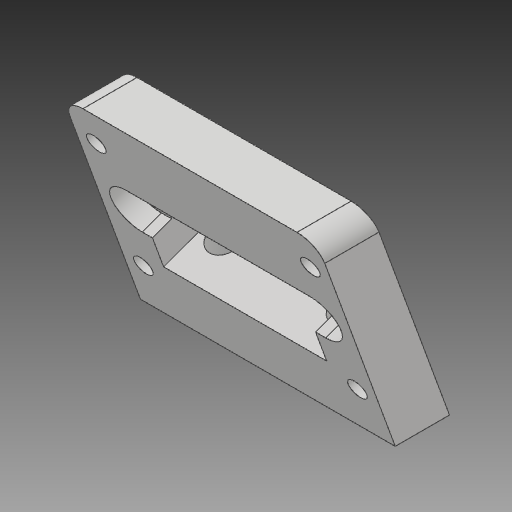
# Autodesk Inventor part: Kamerahalter Vorne geneigt
Saved by Autodesk Inventor 2019.4 (Build 234330000, 330)
## iProperties
Part Number: Kamerahalter Vorne geneigt
Material: Generisch
Document SubType Name: Modeling
Designer: rYan
Density: 1 g/cm^3
Appearance: Vorgabe
Mass: 1.96506 g
Surface Area: 17.9006 cm^2
Volume: 1.96506 cm^3
Author: rYan
Autodesk Inventor part; units mm, degrees
ref_plane "YZ Plane" through (0, 0, 0) normal (1, 0, 0) x (0, 1, 0)
ref_plane "XZ Plane" through (0, 0, 0) normal (0, 1, 0) x (-1, 0, 0)
ref_plane "XY Plane" through (0, 0, 0) normal (0, 0, 1) x (1, 0, 0)
sketch "Skizze1" plane through (0, 0, 0) normal (1, 0, 0) x (0, 1, 0)
  line L0 (2.6604, 0) -> (-2.6604, 0)
  line L1 (-2.6604, 0) -> (-10.3038, 21)
  line L2 (-10.3038, 21) -> (-4.9829, 21)
  line L3 (-4.9829, 21) -> (2.6604, 0)
  point P0 (0, 0)
  point P1 (0, 0)
  dimension "d1" = 21
  dimension "d2" = 70
  dimension "d33" = 5
  constraints: 8 end point, 2 parallel, 1 coincident, 1 horizontal, 1 midpoint
  measures "d1" distance between parallel lines of L0 L2
  measures "d2" angle of L0 L1
  measures "d33" distance between parallel lines of L3 L1
extrude "Extrusion1" add sketch "Skizze1" along normal mid plane 25
sketch "Skizze3" plane through (-12.5, -2.6604, 0) normal (0, -0.9396926, -0.3420201) x (1, 0, 0)
  line L0 (25, 0) -> (0, 0) projected
  line L1 (25, 22.3477) -> (25, 0) projected
  line L2 (25, 22.3477) -> (0, 22.3477) projected
  line L3 (0, 0) -> (0, 22.3477) projected
  line L4 (3.5, 12) -> (21.5, 12) construction
  line L5 (3.5, 9.7) -> (21.5, 9.7)
  line L6 (21.5, 14.3) -> (3.5, 14.3)
  arc A0 (3.5, 14.3) -> (3.5, 9.7) centre (3.5, 12) ccw
  arc A1 (21.5, 9.7) -> (21.5, 14.3) centre (21.5, 12) ccw
  line L7 (12.5, 22.3477) -> (12.5, 0) construction
  point P0 (12.5, -0.9099)
  point P1 (12.5, 12)
  dimension "d10" = 4.6
  dimension "d11" = 18
  dimension "d12" = 12
  constraints: 10 end point, 4 point on circle, 4 tangent, 3 midpoint, 2 centre point, 1 horizontal, 1 parallel, 1 point on line
  measures "d10" diameter of A1
  measures "d11" distance of L4.start L4.end
  measures "d12" distance between parallel lines of L0 L4
extrude "Extrusion3" cut sketch "Skizze3" against normal blind 2 contours A0 L6 A1 L5
sketch "Skizze4" plane through (-12.5, -2.6604, 0) normal (0, -0.9396926, -0.3420201) x (1, 0, 0)
  line L0 (2, 18.5) -> (23, 18.5) construction
  line L1 (23, 18.5) -> (23, 5) construction
  line L2 (23, 5) -> (2, 5) construction
  line L3 (2, 5) -> (2, 18.5) construction
  line L4 (3.5, 14.3) -> (21.5, 14.3) projected
  arc A0 (21.5, 9.7) -> (21.5, 14.3) centre (21.5, 12) ccw projected
  line L5 (21.5, 9.7) -> (3.5, 9.7) projected
  arc A1 (3.5, 14.3) -> (3.5, 9.7) centre (3.5, 12) ccw projected
  line L6 (25, 0) -> (0, 0) projected
  line L7 (25, 22.3477) -> (25, 0) projected
  line L8 (25, 22.3477) -> (0, 22.3477) projected
  line L9 (0, 0) -> (0, 22.3477) projected
  line L10 (25, 22.3477) -> (0, 22.3477) construction
  line L11 (12.5, 22.3477) -> (12.5, 0) construction
  line L12 (25, 0) -> (0, 0) construction
  point P0 (12.5, -0.9099)
  dimension "d15" = 21
  dimension "d16" = 13.5
  dimension "d34" = 7
  constraints: 10 end point, 4 coincident, 2 midpoint, 2 parallel, 1 horizontal, 1 perpendicular, 1 other
  measures "d15" distance of L0.start L0.end
  measures "d16" distance of L2.end L0.start
  measures "d34" distance from line of L2 A1.centre
hole "Bohrung1" at (-10.5, -8.9878, 17.3843) at (10.5, -8.9878, 17.3843) at (10.5, -4.3705, 4.6985) at (-10.5, -4.3705, 4.6985) direction (0, 0.9396926, 0.3420201) diameter 1.85 end through all
sketch "Skizze5" plane through (12.5, 2.6604, 0) normal (0, 0, -1) x (-1, 0, 0)
  line L0 (25, 0) -> (0, 0) projected
  line L1 (0, -5.3209) -> (0, 0) projected
  line L2 (0, -5.3209) -> (25, -5.3209) projected
  line L3 (25, 0) -> (25, -5.3209) projected
  line L4 (0, -5.3209) -> (0, 0) construction
  line L5 (25, 0) -> (25, -5.3209) construction
  line L6 (0, -3.6604) -> (25, -3.6604) construction
  line L7 (25, 0) -> (0, 0) construction
  line L8 (12.5, 0) -> (12.5, -5.3209) construction
  point P0 (12.5, -2.6604)
  point P1 (6.5, -3.6604)
  point P2 (18.5, -3.6604)
  dimension "d25" = 12
  dimension "d43" = 1
  constraints: 4 end point, 4 point on line, 2 midpoint, 1 symmetric about line
  measures "d25" distance of point (18.5, -3.66) point (6.5, -3.66)
  measures "d43" distance from line of point (12.5, -2.66) L6
hole "Bohrung2" at (6, -1, 0) at (-6, -1, 0) direction (0, 0, 1) diameter 2.75 end through all
sketch "Skizze6" plane through (-12.5, -2.6604, 0) normal (0, -0.9396926, -0.3420201) x (1, 0, 0)
  line L0 (21.5, 9.7) -> (3.5, 9.7) projected
  arc A0 (21.5, 9.7) -> (21.5, 14.3) centre (21.5, 12) ccw projected
  line L1 (3.5, 14.3) -> (21.5, 14.3) projected
  arc A1 (3.5, 14.3) -> (3.5, 9.7) centre (3.5, 12) ccw projected
  line L2 (3.5, 14.3) -> (21.5, 14.3) projected
  line L3 (4.5, 14.3) -> (20.5, 14.3)
  line L4 (20.5, 14.3) -> (20.5, 6.5)
  line L5 (20.5, 6.5) -> (4.5, 6.5)
  line L6 (4.5, 6.5) -> (4.5, 14.3)
  line L7 (21.5, 9.7) -> (3.5, 9.7) construction
  line L8 (12.5, 9.7) -> (12.5, 14.3) construction
  point P0 (12.5, -0.9099)
  dimension "d35" = 16
  dimension "d36" = 7.8
  constraints: 10 end point, 2 midpoint, 2 parallel, 2 perpendicular, 1 horizontal, 1 point on line, 1 other
  measures "d35" distance of L4.end L5.end
  measures "d36" distance of L3.end L4.end
extrude "Extrusion4" cut sketch "Skizze6" against normal through all contours L4 L5 L6 L0 | L0 L6 L1 L4
fillet "Rundung1" radius 2 2 edges at (-12.5, -7.6434, 21) (12.5, -7.6434, 21)
chamfer "Fase1" distance 0.3 angle 45 4 edges at (10.5, 0.0115, 7.2778) (10.5, -4.6057, 19.9636) (-10.5, -4.6057, 19.9636) (-10.5, 0.0115, 7.2778)
sketch "Skizze7" plane through (-12.5, 2.6604, 0) normal (0, 0.9396926, 0.3420201) x (1, 0, 0)
  circle A0 centre (2, -20.3199) radius 1.225 projected
  circle A1 centre (23, -6.8199) radius 1.225 projected
  ellipse E0 centre (23, -20.2194) end of major axis (23, -22.3477) minor radius 2 (23, -22.3477) -> (25, -20.2194) ccw projected
  line L0 (25, 0) -> (25, -20.2194) projected
  line L1 (0, 0) -> (25, 0) projected
  line L2 (0, -20.2194) -> (0, 0) projected
  ellipse E1 centre (2, -20.2194) end of major axis (2, -22.3477) minor radius 2 (0, -20.2194) -> (2, -22.3477) ccw projected
  line L3 (23, -22.3477) -> (2, -22.3477) projected
  line L4 (19.6075, -8.3199) -> (20.5, -8.3199) projected
  line L5 (20.5, -8.3199) -> (20.5, -16.1199) projected
  line L6 (20.5, -16.1199) -> (4.5, -16.1199) projected
  line L7 (4.5, -16.1199) -> (4.5, -8.3199) projected
  line L8 (4.5, -8.3199) -> (5.3925, -8.3199) projected
  ellipse E2 centre (6.5, -10.7024) end of major axis (6.5, -6.6822) minor radius 1.375 (7.6075, -8.3199) -> (5.3925, -8.3199) ccw projected
  line L9 (7.6075, -8.3199) -> (17.3925, -8.3199) projected
  ellipse E3 centre (18.5, -10.7024) end of major axis (18.5, -6.6822) minor radius 1.375 (19.6075, -8.3199) -> (17.3925, -8.3199) ccw projected
  circle A2 centre (23, -20.3199) radius 1.225 projected
  circle A3 centre (2, -6.8199) radius 1.225 projected
  line L10 (13, -17.5949) -> (12, -17.5949)
  line L11 (12, -17.5949) -> (12, -20.5949)
  line L12 (12, -20.5949) -> (13, -20.5949)
  line L13 (13, -20.5949) -> (13, -17.5949)
  line L14 (13, -17.5949) -> (12, -20.5949) construction
  line L15 (12, -17.5949) -> (13, -20.5949) construction
  point P0 (12.5, -0.9099)
  point P1 (12.5, -19.0949)
  dimension "d44" = 1
  dimension "d45" = 3
  constraints: 12 end point, 2 midpoint, 2 parallel, 1 horizontal, 1 perpendicular, 4 other
  measures "d44" distance of L12.end L11.end
  measures "d45" distance of L11.end L10.end
extrude "Extrusion5" cut sketch "Skizze7" against normal blind 0.2 contours L13 L12 L11 L10
